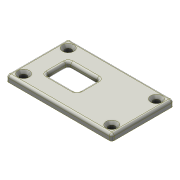
# Autodesk Inventor part: крышка корпус
Saved by Autodesk Inventor 2021 (Build 250183000, 183)
## iProperties
Created: 2023-02-07
Part Number: крышка корпус
Material: Типовые
Document SubType Name: Modeling
Designer: Tasya
Density: 1 g/cm^3
Appearance: Гладкий - слоновая кость
Mass: 2.25476 g
Surface Area: 22.6949 cm^2
Volume: 2.25476 cm^3
Author: Tasya
Autodesk Inventor part; units mm, degrees
ref_plane "YZ Plane" through (0, 0, 0) normal (1, 0, 0) x (0, 1, 0)
ref_plane "XZ Plane" through (0, 0, 0) normal (0, 1, 0) x (-1, 0, 0)
ref_plane "XY Plane" through (0, 0, 0) normal (0, 0, 1) x (1, 0, 0)
sketch "Эскиз1" plane through (0, 0, 0) normal (0, 1, 0) x (-1, 0, 0)
  line L0 (-7.75, 6) -> (7.75, 6) construction
  line L1 (7.75, 6) -> (7.75, -6) construction
  line L2 (7.75, -6) -> (-7.75, -6) construction
  line L3 (-7.75, -6) -> (-7.75, 6) construction
  line L4 (-7.75, 6) -> (7.75, -6) construction
  line L5 (7.75, 6) -> (-7.75, -6) construction
  line L6 (14.25, 12.5) -> (-14.25, 12.5)
  line L7 (-14.25, 12.5) -> (-14.25, -12.5) construction
  line L8 (-14.25, -12.5) -> (14.25, -12.5)
  line L9 (14.25, -12.5) -> (14.25, 12.5)
  line L10 (8.75, 7) -> (-8.75, 7) construction
  line L11 (-8.75, 7) -> (-8.75, -7) construction
  line L12 (-8.75, -7) -> (8.75, -7) construction
  line L13 (8.75, -7) -> (8.75, 7) construction
  line L14 (6.25, 4.5) -> (-6.25, 4.5)
  line L15 (-6.25, 4.5) -> (-6.25, -4.5)
  line L16 (-6.25, -4.5) -> (6.25, -4.5)
  line L17 (6.25, -4.5) -> (6.25, 4.5)
  line L18 (-14.25, -12.5) -> (-28.25, -12.5)
  line L19 (-28.25, -12.5) -> (-28.25, 12.5)
  line L20 (-28.25, 12.5) -> (-14.25, 12.5)
  line L21 (-14.25, 12.5) -> (-14.25, -12.5) construction
  point P0 (0, 0)
  point P1 (-14.25, 12.5)
  dimension "d2" = 15.5
  dimension "d3" = 12
  dimension "d20" = 25
  dimension "d21" = 14
  dimension "d22" = 1.5
  dimension "d42" = 42.5
  constraints: 44 end point, 10 parallel, 5 perpendicular, 2 horizontal, 2 midpoint, 1 collinear, 9 other
  measures "d2" distance of L1.end L2.end
  measures "d3" distance of L0.end L1.end
  measures "d20" distance of L8.end L6.start
  measures "d21" distance of L12.end L10.start
  measures "d22" distance between parallel lines of L1 L17
  measures "d42" distance between parallel lines of L9 L19
extrude "Выдавливание1" add sketch "Эскиз1" along normal blind 2.5
sketch "Эскиз2" plane through (0, 2.5, 0) normal (0, 1, 0) x (1, 0, 0)
  line L0 (8.75, 7) -> (-8.75, 7) construction
  line L1 (-8.75, 7) -> (-8.75, -7) construction
  line L2 (-8.75, -7) -> (8.75, -7) construction
  line L3 (8.75, -7) -> (8.75, 7) construction
  line L4 (8.75, 7) -> (-8.75, -7) construction
  line L5 (-8.75, 7) -> (8.75, -7) construction
  line L6 (-14.25, -12.5) -> (28.25, -12.5) construction
  line L7 (6.25, -4.5) -> (-6.25, -4.5) construction
  line L8 (-14.25, -12.5) -> (-6.25, -4.5) construction
  circle A0 centre (-10.75, -9) radius 1.35 construction
  point P0 (0, 0)
  point P1 (-10.75, 9)
  point P2 (24.75, -9)
  point P3 (24.75, 9)
  dimension "d23" = 14
  dimension "d24" = 17.5
  dimension "d25" = 2.7
  dimension "d27" = 2
  dimension "d30" = 18
  dimension "d33" = 35.5
  constraints: 14 end point, 2 horizontal, 2 midpoint, 2 parallel, 1 centre point, 1 coincident, 1 perpendicular, 1 point on line, 1 vertical, 3 other
  measures "d23" distance of L0.end L1.end
  measures "d24" distance of L0.start L0.end
  measures "d25" diameter of A0
  measures "d27" distance from line of L2 A0.centre
  measures "d30" distance of point (-10.75, -9) point (-10.75, 9)
  measures "d33" distance of point (-10.75, -9) point (24.75, -9)
hole "Отверстие1" at (-10.75, 2.5, -9) at (24.75, 2.5, -9) at (24.75, 2.5, 9) at (-10.75, 2.5, 9) direction (0, -1, 0) diameter 2.6 end through all countersink diameter 4.6 countersink angle 90 clearance for "с потайной головкой ГОСТ 12876-67" size "M2" standard "ГОСТ"
fillet "Сопряжение5" radius 1 20 edges at (-14.25, 2.5, 0) (7, 2.5, -12.5) (-14.25, 1.25, -12.5) (7, 2.5, 12.5) (-14.25, 1.25, 12.5) (-6.25, 2.5, 0) (-6.25, 1.25, -4.5) (0, 2.5, -4.5) (-6.25, 0, 0) (0, 0, -4.5) (6.25, 1.25, 4.5) (6.25, 2.5, 0) (6.25, 0, 0) (6.25, 1.25, -4.5) (-6.25, 1.25, 4.5) (0, 2.5, 4.5) (0, 0, 4.5) (28.25, 1.25, 12.5) (28.25, 2.5, 0) (28.25, 1.25, -12.5)
equation "\"d30\" = d23 + 2 * d27"
